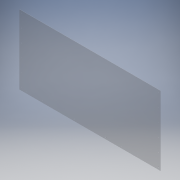
# Autodesk Inventor part: Long Wall
Saved by Autodesk Inventor 2017 (Build 210142000, 142)
## iProperties
Created: 2017-01-16
Part Number: Long Wall
Material: Polycarbonate, Clear
Document SubType Name: Modeling
Designer: Ben
Density: 1.2 g/cm^3
Appearance: Polycarbonate - Clear
Mass: 566.199 g
Surface Area: 5980.63 cm^2
Volume: 471.832 cm^3
Author: Ben
Autodesk Inventor part; units mm, degrees
ref_plane "YZ Plane" through (0, 0, 0) normal (1, 0, 0) x (0, 1, 0)
ref_plane "XZ Plane" through (0, 0, 0) normal (0, 1, 0) x (-1, 0, 0)
ref_plane "XY Plane" through (0, 0, 0) normal (0, 0, 1) x (1, 0, 0)
sketch "Sketch1" plane through (0, 0, 0) normal (0, 0, 1) x (1, 0, 0)
  line L0 (0, 0) -> (762, 0)
  line L1 (762, 0) -> (762, 368.3)
  line L2 (762, 368.3) -> (0, 368.3)
  line L3 (0, 368.3) -> (0, 0)
  line L4 (752.475, 368.3) -> (752.475, 0) construction
  line L5 (762, 184.15) -> (0, 184.15) construction
  line L6 (381, 368.3) -> (381, 0) construction
  line L7 (762, 9.525) -> (0, 9.525) construction
  circle A0 centre (381, 9.525) radius 1.5875
  circle A1 centre (295.275, 9.525) radius 1.5875
  circle A2 centre (209.55, 9.525) radius 1.5875
  circle A3 centre (123.825, 9.525) radius 1.5875
  circle A4 centre (38.1, 9.525) radius 1.5875
  circle A5 centre (466.725, 9.525) radius 1.5875
  circle A6 centre (552.45, 9.525) radius 1.5875
  circle A7 centre (638.175, 9.525) radius 1.5875
  circle A8 centre (723.9, 9.525) radius 1.5875
  circle A9 centre (752.475, 184.15) radius 1.5875
  circle A10 centre (752.475, 107.95) radius 1.5875
  circle A11 centre (752.475, 31.75) radius 1.5875
  circle A12 centre (752.475, 260.35) radius 1.5875
  circle A13 centre (752.475, 184.15) radius 1.5875
  circle A14 centre (752.475, 107.95) radius 1.5875
  circle A15 centre (752.475, 336.55) radius 1.5875
  circle A16 centre (752.475, 260.35) radius 1.5875
  circle A17 centre (752.475, 184.15) radius 1.5875
  line L8 (9.525, 368.3) -> (9.525, 0) construction
  circle A18 centre (9.525, 184.15) radius 1.5875
  circle A19 centre (9.525, 107.95) radius 1.5875
  circle A20 centre (9.525, 31.75) radius 1.5875
  circle A21 centre (9.525, 260.35) radius 1.5875
  circle A22 centre (9.525, 184.15) radius 1.5875
  circle A23 centre (9.525, 107.95) radius 1.5875
  circle A24 centre (9.525, 336.55) radius 1.5875
  circle A25 centre (9.525, 260.35) radius 1.5875
  circle A26 centre (9.525, 184.15) radius 1.5875
  dimension "d0" = 762
  dimension "d1" = 368.3
  dimension "d12" = 9.525
  dimension "d13" = 9.525
  dimension "d16" = 85.725
  dimension "d23" = 85.725
  dimension "d28" = 3.175
  dimension "d31" = 76.2
  dimension "d34" = 76.2
  constraints: 27 centre point, 18 end point, 11 symmetric about line, 7 midpoint, 5 point on line, 3 horizontal, 3 parallel, 2 perpendicular, 2 vertical, 1 equal radius, 41 other
  measures "d0" distance of L0.start L0.end
  measures "d1" distance of L2.end L0.start
  measures "d12" distance between parallel lines of L4 L1
  measures "d13" distance between parallel lines of L7 L0
  measures "d16" distance of A0.centre A1.centre
  measures "d23" distance of A0.centre A5.centre
  measures "d28" diameter of A8
  measures "d31" distance of A9.centre A10.centre
  measures "d34" distance of A9.centre A12.centre
extrude "Extrusion1" add sketch "Sketch1" along normal blind 1.5875
equation "\"d13\" = d12"
body "Solid1"
